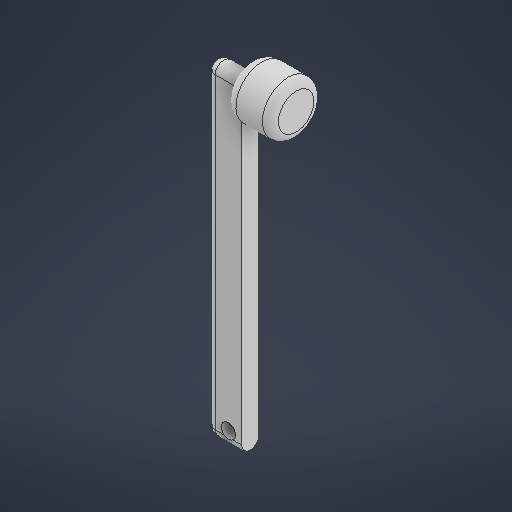
# Autodesk Inventor part: braço
Saved by Autodesk Inventor 2027 (Build 310192060, 192F)
## iProperties
Created: 2026-10-07
Part Number: braço
Material: Genérico
Document SubType Name: Modeling
Designer: guisg
Density: 1 g/cm^3
Appearance: Padrão
Author: guisg
Autodesk Inventor part; units mm, degrees
ref_plane "YZ Plane" through (0, 0, 0) normal (1, 0, 0) x (0, 1, 0)
ref_plane "XZ Plane" through (0, 0, 0) normal (0, 1, 0) x (-1, 0, 0)
ref_plane "XY Plane" through (0, 0, 0) normal (0, 0, 1) x (1, 0, 0)
sketch "Esboço1" plane through (0, 0, 0) normal (1, 0, 0) x (0, 1, 0)
  circle A0 centre (0, 0) radius 22.5
  dimension "d0" = 45
  constraints: 1 centre point, 1 coincident
  measures "d0" diameter of A0
extrude "Extrusão1" add sketch "Esboço1" along normal blind 40
fillet "Arredondamento1" radius 10 1 edges at (0, -22.5, 0)
sketch "Esboço2" plane through (0, 0, 0) normal (-1, 0, 0) x (0, 0, 1)
  line L0 (0, 0) -> (0, -268) construction
  line L1 (-7.5, 0) -> (-7.5, -268)
  line L2 (7.5, -268) -> (7.5, 0)
  arc A0 (7.5, 0) -> (-7.5, 0) centre (0, 0) ccw
  arc A1 (-7.5, -268) -> (7.5, -268) centre (0, -268) ccw
  point P0 (0, -134)
  dimension "d5" = 15
  constraints: 8 end point, 4 point on circle, 4 tangent, 2 centre point, 1 midpoint, 1 parallel, 1 vertical
  measures "d5" diameter of A1
extrude "Extrusão2" add sketch "Esboço2" along normal blind 30
fillet "Arredondamento2" radius 7 5 edges at (-30, -134, 7.5) (-30, 7.5, 0) (-30, -134, -7.5) (-30, -275.5, 0) (40, -22.5, 0)
sketch "Esboço3" plane through (0, -268, 7.5) normal (0, 0, 1) x (1, 0, 0)
  circle A0 centre (-11.5, 5) radius 6.25
  point P0 (0, 268)
  constraints: 1 centre point
extrude "Extrusão3" cut sketch "Esboço3" against normal blind 30
